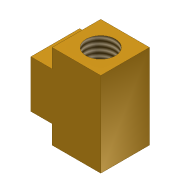
# Autodesk Inventor part: 2203P-2
Saved by Autodesk Inventor 2014 SP1 (Build 180222100, 222)
## iProperties
Category: Pneumatics
Shininess: 64.0
Length Units: 11272
Angle Units: 11279
Time Units: 11290
Mass Units: 11283
Length Display Precision: 3
Angle Display Precision: 2
Compacted: True
Document SubType Name: Modeling
Created: 2005-01-08
Manufacturer: Standard
Standards Organization: Custom
Vendor: Parker
Project: FIRST
Description: Union Tee
Part Number: 2203P-2
Density: 1 g/cm^3
Material: Generic
Appearance: Brass - Satin
Mass: 4.60615 g
Surface Area: 30.172 cm^2
Volume: 4.60615 cm^3
Density: 0.0
Volumn: 0.0
Area: 0.0
PropertySet Name: Model Information
Control State: 0
Master: False
Checked Out: False
Title: Union Tee
Author: Autodesk, Inc.
Autodesk Inventor part; units mm, degrees
ref_plane "YZ Plane" through (0, 0, 0) normal (1, 0, 0) x (0, 1, 0)
ref_plane "XZ Plane" through (0, 0, 0) normal (0, 1, 0) x (-1, 0, 0)
ref_plane "XY Plane" through (0, 0, 0) normal (0, 0, 1) x (1, 0, 0)
sketch "Sketch1" plane through (0, 0, 0) normal (0, 0, 1) x (1, 0, 0)
  line L0 (-7.3025, 7.3025) -> (7.3025, 7.3025)
  line L1 (7.3025, 7.3025) -> (7.3025, -7.3025)
  line L2 (7.3025, -7.3025) -> (-7.3025, -7.3025)
  line L3 (-7.3025, -7.3025) -> (-7.3025, 7.3025)
  point P0 (0, 0)
  point P1 (0, 7.3025)
  point P2 (-7.3025, 0)
  dimension "d0" = 14.605
  dimension "d1" = 14.605
  constraints: 8 end point, 2 midpoint, 2 parallel, 1 horizontal, 1 horizontal alignment, 1 perpendicular, 1 vertical alignment
  measures "d0" distance between parallel lines of L0 L2
  measures "d1" distance between parallel lines of L3 L1
extrude "Extrusion1" add sketch "Sketch1" along normal mid plane 25.4
sketch "Sketch2" plane through (-7.3025, -7.3025, 12.7) normal (-1, 0, 0) x (0, 0, 1)
  line L0 (0, 0) -> (0, 14.605) projected
  line L1 (-25.4, 14.605) -> (0, 14.605) projected
  line L2 (-25.4, 14.605) -> (-25.4, 0) projected
  line L3 (0, 0) -> (-25.4, 0) projected
  line L4 (-19.812, 14.605) -> (-5.588, 14.605)
  line L5 (-5.588, 14.605) -> (-5.588, 0)
  line L6 (-5.588, 0) -> (-19.812, 0)
  line L7 (-19.812, 0) -> (-19.812, 14.605)
  point P0 (-12.7, 0)
  dimension "d4" = 14.224
  constraints: 8 end point, 2 midpoint, 2 parallel, 2 point on line, 1 horizontal, 1 perpendicular
  measures "d4" distance between parallel lines of L5 L7
extrude "Extrusion2" add sketch "Sketch2" along normal blind 6.35 contours L3 L7 L1 L5
sketch "Sketch3" plane through (0, 0, -12.7) normal (0, 0, -1) x (-1, 0, 0)
  line L0 (7.3025, 7.3025) -> (7.3025, -7.3025) projected
  line L1 (-7.3025, 7.3025) -> (7.3025, 7.3025) projected
  line L2 (-7.3025, -7.3025) -> (-7.3025, 7.3025) projected
  line L3 (7.3025, -7.3025) -> (-7.3025, -7.3025) projected
  circle A0 centre (0, 0) radius 4.3815
  dimension "d7" = 8.763
  constraints: 1 centre point
  measures "d7" diameter of A0
extrude "Extrusion3" cut sketch "Sketch3" against normal through all contours A0
sketch "Sketch4" plane through (-13.6525, -7.3025, 12.7) normal (-1, 0, 0) x (0, 0, 1)
  circle A0 centre (-12.7, 7.3025) radius 4.3815
  line L0 (-19.812, 0) -> (-19.812, 14.605) projected
  line L1 (0, 0) -> (-25.4, 0) projected
  line L2 (-19.812, 14.605) -> (-5.588, 14.605) projected
  line L3 (-19.812, 0) -> (-19.812, 14.605) projected
  line L4 (-5.588, 0) -> (-19.812, 0) projected
  line L5 (-5.588, 14.605) -> (-5.588, 0) projected
  point P0 (-12.7, 14.605)
  point P1 (-19.812, 7.3025)
  dimension "d10" = 8.763
  constraints: 2 midpoint, 1 centre point, 1 horizontal alignment, 1 vertical alignment
  measures "d10" diameter of A0
extrude "Extrusion4" cut sketch "Sketch4" against normal blind 13.7414 contours A0
thread "Thread1" size "3/8-16 UNC" class "1B" standard "ANSI Unified Screw Threads" length 8.89
thread "Thread2" size "3/8-16 UNC" class "1B" standard "ANSI Unified Screw Threads" length 8.89
thread "Thread3" size "3/8-16 UNC" class "1B" standard "ANSI Unified Screw Threads" length 8.89
equation "\"d0\" = d1"
body "Solid1"
